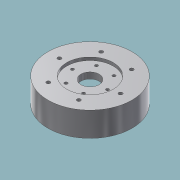
# Autodesk Inventor part: Spur Gear2
Saved by Autodesk Inventor 2017 SP1 (Build 210196100, 196)
## iProperties
Created: 2018-10-09
Part Number: Spur Gear2
Material: ABS Plastic
Document SubType Name: Modeling
Designer: Zach
Categories: <?xml version="1.0" encoding="UTF-16"?> <MemberInstance><Categories><FamilyTemplate><FamilyTemplateParameter ValueType="xs:double" Id="1" ObjectReferenceKey="da_z" ObjectType="kUserParameterObject"/><FamilyTemplateParameter ValueType="xs:double" Id="2" ObjectReferenceKey="da_b" ObjectType="kUserParameterObject"/><FamilyTemplateParameter ValueType="xs:double" Id="3" ObjectReferenceKey="da_beta" ObjectType="kUserParameterObject"/><FamilyTemplateParameter ValueType="xs:double" Id="4" ObjectReferenceKey="da_da" ObjectType="kUserParameterObject"/><FamilyTemplateParameter ValueType="xs:double" Id="5" ObjectReferenceKey="da_aw" ObjectType="kUserParameterObject"/><FamilyTemplateParameter ValueType="xs:string" Id="6" ObjectReferenceKey="EAIAABAAAACIAQAAAAAAAIAAAAAAAAAA" ObjectType="83910656" SubObjectId="SurfaceGeometry"/></FamilyTemplate><ParamToTemplateMap><ParamToTemplate CategoryParameter="//CategoryParameter[@InternalName='046C89C9-8512-4d59-83FE-43B91F4F132A']" TemplateParameter="1"/><ParamToTemplate CategoryParameter="//CategoryParameter[@InternalName='2552DF32-E462-4b46-AEBF-C6C7768E72AC']" TemplateParameter="2"/><ParamToTemplate CategoryParameter="//CategoryParameter[@InternalName='C9EE641D-15FC-4fae-A226-E94C4372FDD7']" TemplateParameter="3"/><ParamToTemplate><ParamToTemplate CategoryParameter="//CategoryParameter[@InternalName='00B6519A-459B-49c7-AD84-2E56D39A5744']" ConstantValue="0.000000"/></ParamToTemplate><ParamToTemplate><ParamToTemplate CategoryParameter="//CategoryParameter[@InternalName='04B31F0E-C7A6-4894-AA32-9629BEFACF47']" ConstantValue="1.000000"/></ParamToTemplate><ParamToTemplate><ParamToTemplate CategoryParameter="//CategoryParameter[@InternalName='43CBEC2E-7847-49e7-A936-2F7889FCB2D9']" ConstantValue="0.250000"/></ParamToTemplate><ParamToTemplate><ParamToTemplate CategoryParameter="//CategoryParameter[@InternalName='B1EFC894-105D-4ebd-86BF-FA20ED196853']" ConstantValue="0.350000"/></ParamToTemplate><ParamToTemplate><ParamToTemplate CategoryParameter="//CategoryParameter[@InternalName='51175063-3D10-4879-93E8-6246FE8B403D']" ConstantValue="2060000000.000000"/></ParamToTemplate><ParamToTemplate><ParamToTemplate CategoryParameter="//CategoryParameter[@InternalName='A3A52E27-4454-46a9-B0BD-C932399B70AF']" ConstantValue="0.300000"/></ParamToTemplate><ParamToTemplate><ParamToTemplate CategoryParameter="//CategoryParameter[@InternalName='91B76062-C214-41d9-B1B9-14D2AB99603D']" ConstantValue="0.200000"/></ParamToTemplate><ParamToTemplate><ParamToTemplate CategoryParameter="//CategoryParameter[@InternalName='374E806E-8B8A-4dda-A9AA-1039D6500AD2']" ConstantValue="5.000000"/></ParamToTemplate><ParamToTemplate><ParamToTemplate CategoryParameter="//CategoryParameter[@InternalName='2D373A89-B862-43d6-8D0B-0CBF12AB9F6C']" ConstantValue="0.392699"/></ParamToTemplate><ParamToTemplate CategoryParameter="//CategoryParameter[@InternalName='37777632-D6A2-4fac-9D53-DB8ACD95C989']" TemplateParameter="4"/><ParamToTemplate CategoryParameter="//CategoryParameter[@InternalName='FD1017F1-B727-4f7e-9707-0F86F1FF9423']" TemplateParameter="5"/><ParamToTemplate><ParamToTemplate CategoryParameter="//CategoryParameter[@InternalName='9E1B4470-B2D3-4ff1-B813-535BB4CDF51A']" ConstantValue="3520000.000000"/></ParamToTemplate><ParamToTemplate><ParamToTemplate CategoryParameter="//CategoryParameter[@InternalName='F8452263-BFF6-458c-9FB1-07C4B99E95CD']" ConstantValue="11400000.000000"/></ParamToTemplate><ParamToTemplate><ParamToTemplate CategoryParameter="//CategoryParameter[@InternalName='3E3BB259-FD49-497f-8171-6EBC954A3479']" ConstantValue="2.000000"/></ParamToTemplate><ParamToTemplate CategoryParameter="//CategoryParameter[@InternalName='27C3BAF2-7550-4e4b-AE2C-0DB134B7D9B7']" TemplateParameter="6"/></ParamToTemplateMap><Category DisplayName="Gear" InternalName="DC85795E-93AB-48d5-8EEE-5A27447B64BD" Mnemonic="Gear"><CategoryParameter DisplayName="z" InternalName="046C89C9-8512-4d59-83FE-43B91F4F132A" Mnemonic="z"/><CategoryParameter DisplayName="b" InternalName="2552DF32-E462-4b46-AEBF-C6C7768E72AC" Mnemonic="b"/><CategoryParameter DisplayName="||b|" InternalName="C9EE641D-15FC-4fae-A226-E94C4372FDD7" Mnemonic="beta"/><CategoryParameter DisplayName="x" InternalName="00B6519A-459B-49c7-AD84-2E56D39A5744" Mnemonic="x"/><CategoryParameter DisplayName="a*" InternalName="04B31F0E-C7A6-4894-AA32-9629BEFACF47" Mnemonic="a"/><CategoryParameter DisplayName="c*" InternalName="43CBEC2E-7847-49e7-A936-2F7889FCB2D9" Mnemonic="c"/><CategoryParameter DisplayName="r|.f|*" InternalName="B1EFC894-105D-4ebd-86BF-FA20ED196853" Mnemonic="rf"/><CategoryParameter DisplayName="E" InternalName="51175063-3D10-4879-93E8-6246FE8B403D" Mnemonic="E"/><CategoryParameter DisplayName="||m|" InternalName="A3A52E27-4454-46a9-B0BD-C932399B70AF" Mnemonic="mi"/><Category DisplayName="SpurGear" InternalName="26C5A22E-A91E-4dfd-A3B3-23CCAFAE1764" Mnemonic="SpurGear"><CategoryParameter DisplayName="m" InternalName="91B76062-C214-41d9-B1B9-14D2AB99603D" Mnemonic="m"/><CategoryParameter DisplayName="P" InternalName="374E806E-8B8A-4dda-A9AA-1039D6500AD2" Mnemonic="PP"/><CategoryParameter DisplayName="||a|" InternalName="2D373A89-B862-43d6-8D0B-0CBF12AB9F6C" Mnemonic="alpha"/><CategoryParameter DisplayName="d|.a|" InternalName="37777632-D6A2-4fac-9D53-DB8ACD95C989" Mnemonic="da"/><CategoryParameter DisplayName="a|.w|" InternalName="FD1017F1-B727-4f7e-9707-0F86F1FF9423" Mnemonic="aw"/><CategoryParameter DisplayName="||s||.Flim|" InternalName="9E1B4470-B2D3-4ff1-B813-535BB4CDF51A" Mnemonic="sFlim"/><CategoryParameter DisplayName="||s||.Hlim|" InternalName="F8452263-BFF6-458c-9FB1-07C4B99E95CD" Mnemonic="sHlim"/><CategoryParameter DisplayName="type" InternalName="3E3BB259-FD49-497f-8171-6EBC954A3479" Mnemonic="type"/><Category DisplayName="InternalSpurGear" InternalName="7CF704F6-14A9-42f8-93CE-E71DF57C2B55" Mnemonic="InternalSpurGear"><CategoryParameter DisplayName="PitchDiameter" InternalName="27C3BAF2-7550-4e4b-AE2C-0DB134B7D9B7" Mnemonic="IDS_PITCHDIAM"/></Category></Category></Category></Categories></MemberInstance>
Density: 1.06 g/cm^3
Appearance: Smooth - White
CustomPartVersion: 0
Author: Zach
Autodesk Inventor part; units mm, degrees
ref_plane "YZ Plane" through (0, 0, 0) normal (1, 0, 0) x (0, 1, 0)
ref_plane "XZ Plane" through (0, 0, 0) normal (0, 1, 0) x (-1, 0, 0)
ref_plane "XY Plane" through (0, 0, 0) normal (0, 0, 1) x (1, 0, 0)
sketch "Sketch1" plane through (0, 0, 0) normal (0, 0, 1) x (1, 0, 0)
  circle A0 centre (0, 0) radius 68.75
  dimension "d0" = 137.5
  constraints: 1 centre point
  measures "d0" diameter of A0
extrude "Extrusion1" add sketch "Sketch1" along normal blind 10
ref_plane "Work Plane2" through (0, 0, 5) normal (0, 0, 1) x (1, 0, 0)
sketch "Sketch2" plane through (0, 0, 0) normal (0, 0, -1) x (-1, 0, 0)
  circle A0 centre (0, 0) radius 68.75 projected
  circle A1 centre (0, 0) radius 60
  dimension "d3" = 120
  constraints: 1 centre point, 1 coincident
  measures "d3" diameter of A1
surface extrude "Pitch Diameter" sketch "Sketch2" against normal through all shown no curves A1
ref_plane "Work Plane8" through (0, 0, 0) normal (0.9986295, 0.052336, 0) x (0, 0, 1)
ref_plane "Work Plane9" through (0, 0, 0) normal (1, 0, 0) x (0, 1, 0)
spur gear teeth "Spur Gear" teeth 60 pitch diameter 120 tip diameter 116 root diameter 125 face width 10 start plane through (0, 0, 0) normal (0, 0, -1) x (-1, 0, 0)
sketch "Sketch3" plane through (0, 0, 10) normal (0, 0, 1) x (1, 0, 0)
  arc A0 (2.2771, -57.9553) -> (3.7934, -57.8758) centre (0, 0) ccw projected
  arc A1 (0.8181, -62.4946) -> (2.2771, -57.9553) centre (-22.2852, -52.565) ccw projected
  arc A2 (-0.8181, -62.4946) -> (0.8181, -62.4946) centre (0, 0) ccw projected
  arc A3 (-2.2771, -57.9553) -> (-0.8181, -62.4946) centre (22.2852, -52.565) ccw projected
  arc A4 (-3.7934, -57.8758) -> (-2.2771, -57.9553) centre (0, 0) ccw projected
  arc A5 (-5.7189, -62.2378) -> (-3.7934, -57.8758) centre (-27.6576, -49.9476) ccw projected
  arc A6 (-7.3461, -62.0668) -> (-5.7189, -62.2378) centre (0, 0) ccw projected
  arc A7 (-8.3226, -57.3998) -> (-7.3461, -62.0668) centre (16.6686, -54.6065) ccw projected
  arc A8 (-9.8223, -57.1623) -> (-8.3226, -57.3998) centre (0, 0) ccw projected
  arc A9 (-12.1931, -61.2991) -> (-9.8223, -57.1623) centre (-32.7271, -46.783) ccw projected
  arc A10 (-13.7936, -60.9589) -> (-12.1931, -61.2991) centre (0, 0) ccw projected
  arc A11 (-14.2769, -56.2154) -> (-13.7936, -60.9589) centre (10.8693, -56.0497) ccw projected
  arc A12 (-15.7435, -55.8224) -> (-14.2769, -56.2154) centre (0, 0) ccw projected
  arc A13 (-18.5338, -59.6887) -> (-15.7435, -55.8224) centre (-37.438, -43.1058) ccw projected
  arc A14 (-20.09, -59.1831) -> (-18.5338, -59.6887) centre (0, 0) ccw projected
  arc A15 (-20.0748, -54.4151) -> (-20.09, -59.1831) centre (4.951, -56.8788) ccw projected
  arc A16 (-21.4923, -53.871) -> (-20.0748, -54.4151) centre (0, 0) ccw projected
  arc A17 (-24.6715, -57.4245) -> (-21.4923, -53.871) centre (-41.7386, -38.9563) ccw projected
  arc A18 (-26.1662, -56.7589) -> (-24.6715, -57.4245) centre (0, 0) ccw projected
  arc A19 (-25.6527, -52.0186) -> (-26.1662, -56.7589) centre (-1.0216, -57.0847) ccw projected
  arc A20 (-27.0056, -51.3293) -> (-25.6527, -52.0186) centre (0, 0) ccw projected
  arc A21 (-30.5388, -54.531) -> (-27.0056, -51.3293) centre (-45.582, -34.38) ccw projected
  arc A22 (-31.9558, -53.7129) -> (-30.5388, -54.531) centre (0, 0) ccw projected
  arc A23 (-30.9496, -49.0522) -> (-31.9558, -53.7129) centre (-6.983, -56.6652) ccw projected
  arc A24 (-32.2231, -48.2252) -> (-30.9496, -49.0522) centre (0, 0) ccw projected
  arc A25 (-36.0716, -51.0401) -> (-32.2231, -48.2252) centre (-48.926, -29.4271) ccw projected
  arc A26 (-37.3953, -50.0784) -> (-36.0716, -51.0401) centre (0, 0) ccw projected
  arc A27 (-35.9074, -45.5484) -> (-37.3953, -50.0784) centre (-12.8678, -55.6249) ccw projected
  arc A28 (-37.0875, -44.5928) -> (-35.9074, -45.5484) centre (0, 0) ccw projected
  arc A29 (-41.2091, -46.99) -> (-37.0875, -44.5928) centre (-51.734, -24.1517) ccw projected
  arc A30 (-42.425, -45.8952) -> (-41.2091, -46.99) centre (0, 0) ccw projected
  arc A31 (-40.4718, -41.5455) -> (-42.425, -45.8952) centre (-18.6117, -53.9751) ccw projected
  arc A32 (-41.5455, -40.4718) -> (-40.4718, -41.5455) centre (0, 0) ccw projected
  arc A33 (-45.8952, -42.425) -> (-41.5455, -40.4718) centre (-53.9751, -18.6117) ccw projected
  arc A34 (-46.99, -41.2091) -> (-45.8952, -42.425) centre (0, 0) ccw projected
  arc A35 (-44.5928, -37.0875) -> (-46.99, -41.2091) centre (-24.1517, -51.734) ccw projected
  arc A36 (-45.5484, -35.9074) -> (-44.5928, -37.0875) centre (0, 0) ccw projected
  arc A37 (-50.0784, -37.3953) -> (-45.5484, -35.9074) centre (-55.6249, -12.8678) ccw projected
  arc A38 (-51.0401, -36.0716) -> (-50.0784, -37.3953) centre (0, 0) ccw projected
  arc A39 (-48.2252, -32.2231) -> (-51.0401, -36.0716) centre (-29.4271, -48.926) ccw projected
  arc A40 (-49.0522, -30.9496) -> (-48.2252, -32.2231) centre (0, 0) ccw projected
  arc A41 (-53.7129, -31.9558) -> (-49.0522, -30.9496) centre (-56.6652, -6.983) ccw projected
  arc A42 (-54.531, -30.5388) -> (-53.7129, -31.9558) centre (0, 0) ccw projected
  arc A43 (-51.3293, -27.0056) -> (-54.531, -30.5388) centre (-34.38, -45.582) ccw projected
  arc A44 (-52.0186, -25.6527) -> (-51.3293, -27.0056) centre (0, 0) ccw projected
  arc A45 (-56.7589, -26.1662) -> (-52.0186, -25.6527) centre (-57.0847, -1.0216) ccw projected
  arc A46 (-57.4245, -24.6715) -> (-56.7589, -26.1662) centre (0, 0) ccw projected
  arc A47 (-53.871, -21.4923) -> (-57.4245, -24.6715) centre (-38.9563, -41.7386) ccw projected
  arc A48 (-54.4151, -20.0748) -> (-53.871, -21.4923) centre (0, 0) ccw projected
  arc A49 (-59.1831, -20.09) -> (-54.4151, -20.0748) centre (-56.8788, 4.951) ccw projected
  arc A50 (-59.6887, -18.5338) -> (-59.1831, -20.09) centre (0, 0) ccw projected
  arc A51 (-55.8224, -15.7435) -> (-59.6887, -18.5338) centre (-43.1058, -37.438) ccw projected
  arc A52 (-56.2154, -14.2769) -> (-55.8224, -15.7435) centre (0, 0) ccw projected
  arc A53 (-60.9589, -13.7936) -> (-56.2154, -14.2769) centre (-56.0497, 10.8693) ccw projected
  arc A54 (-61.2991, -12.1931) -> (-60.9589, -13.7936) centre (0, 0) ccw projected
  arc A55 (-57.1623, -9.8223) -> (-61.2991, -12.1931) centre (-46.783, -32.7271) ccw projected
  arc A56 (-57.3998, -8.3226) -> (-57.1623, -9.8223) centre (0, 0) ccw projected
  arc A57 (-62.0668, -7.3461) -> (-57.3998, -8.3226) centre (-54.6065, 16.6686) ccw projected
  arc A58 (-62.2378, -5.7189) -> (-62.0668, -7.3461) centre (0, 0) ccw projected
  arc A59 (-57.8758, -3.7934) -> (-62.2378, -5.7189) centre (-49.9476, -27.6576) ccw projected
  arc A60 (-57.9553, -2.2771) -> (-57.8758, -3.7934) centre (0, 0) ccw projected
  arc A61 (-62.4946, -0.8181) -> (-57.9553, -2.2771) centre (-52.565, 22.2852) ccw projected
  arc A62 (-62.4946, 0.8181) -> (-62.4946, -0.8181) centre (0, 0) ccw projected
  arc A63 (-57.9553, 2.2771) -> (-62.4946, 0.8181) centre (-52.565, -22.2852) ccw projected
  arc A64 (-57.8758, 3.7934) -> (-57.9553, 2.2771) centre (0, 0) ccw projected
  arc A65 (-62.2378, 5.7189) -> (-57.8758, 3.7934) centre (-49.9476, 27.6576) ccw projected
  arc A66 (-62.0668, 7.3461) -> (-62.2378, 5.7189) centre (0, 0) ccw projected
  arc A67 (-57.3998, 8.3226) -> (-62.0668, 7.3461) centre (-54.6065, -16.6686) ccw projected
  arc A68 (-57.1623, 9.8223) -> (-57.3998, 8.3226) centre (0, 0) ccw projected
  arc A69 (-61.2991, 12.1931) -> (-57.1623, 9.8223) centre (-46.783, 32.7271) ccw projected
  arc A70 (-60.9589, 13.7936) -> (-61.2991, 12.1931) centre (0, 0) ccw projected
  arc A71 (-56.2154, 14.2769) -> (-60.9589, 13.7936) centre (-56.0497, -10.8693) ccw projected
  arc A72 (-55.8224, 15.7435) -> (-56.2154, 14.2769) centre (0, 0) ccw projected
  arc A73 (-59.6887, 18.5338) -> (-55.8224, 15.7435) centre (-43.1058, 37.438) ccw projected
  arc A74 (-59.1831, 20.09) -> (-59.6887, 18.5338) centre (0, 0) ccw projected
  arc A75 (-54.4151, 20.0748) -> (-59.1831, 20.09) centre (-56.8788, -4.951) ccw projected
  arc A76 (-53.871, 21.4923) -> (-54.4151, 20.0748) centre (0, 0) ccw projected
  arc A77 (-57.4245, 24.6715) -> (-53.871, 21.4923) centre (-38.9563, 41.7386) ccw projected
  arc A78 (-56.7589, 26.1662) -> (-57.4245, 24.6715) centre (0, 0) ccw projected
  arc A79 (-52.0186, 25.6527) -> (-56.7589, 26.1662) centre (-57.0847, 1.0216) ccw projected
  arc A80 (-51.3293, 27.0056) -> (-52.0186, 25.6527) centre (0, 0) ccw projected
  arc A81 (-54.531, 30.5388) -> (-51.3293, 27.0056) centre (-34.38, 45.582) ccw projected
  arc A82 (-53.7129, 31.9558) -> (-54.531, 30.5388) centre (0, 0) ccw projected
  arc A83 (-49.0522, 30.9496) -> (-53.7129, 31.9558) centre (-56.6652, 6.983) ccw projected
  arc A84 (-48.2252, 32.2231) -> (-49.0522, 30.9496) centre (0, 0) ccw projected
  arc A85 (-51.0401, 36.0716) -> (-48.2252, 32.2231) centre (-29.4271, 48.926) ccw projected
  arc A86 (-50.0784, 37.3953) -> (-51.0401, 36.0716) centre (0, 0) ccw projected
  arc A87 (-45.5484, 35.9074) -> (-50.0784, 37.3953) centre (-55.6249, 12.8678) ccw projected
  arc A88 (-44.5928, 37.0875) -> (-45.5484, 35.9074) centre (0, 0) ccw projected
  arc A89 (-46.99, 41.2091) -> (-44.5928, 37.0875) centre (-24.1517, 51.734) ccw projected
  arc A90 (-45.8952, 42.425) -> (-46.99, 41.2091) centre (0, 0) ccw projected
  arc A91 (-41.5455, 40.4718) -> (-45.8952, 42.425) centre (-53.9751, 18.6117) ccw projected
  arc A92 (-40.4718, 41.5455) -> (-41.5455, 40.4718) centre (0, 0) ccw projected
  arc A93 (-42.425, 45.8952) -> (-40.4718, 41.5455) centre (-18.6117, 53.9751) ccw projected
  arc A94 (-41.2091, 46.99) -> (-42.425, 45.8952) centre (0, 0) ccw projected
  arc A95 (-37.0875, 44.5928) -> (-41.2091, 46.99) centre (-51.734, 24.1517) ccw projected
  arc A96 (-35.9074, 45.5484) -> (-37.0875, 44.5928) centre (0, 0) ccw projected
  arc A97 (-37.3953, 50.0784) -> (-35.9074, 45.5484) centre (-12.8678, 55.6249) ccw projected
  arc A98 (-36.0716, 51.0401) -> (-37.3953, 50.0784) centre (0, 0) ccw projected
  arc A99 (-32.2231, 48.2252) -> (-36.0716, 51.0401) centre (-48.926, 29.4271) ccw projected
  arc A100 (-30.9496, 49.0522) -> (-32.2231, 48.2252) centre (0, 0) ccw projected
  arc A101 (-31.9558, 53.7129) -> (-30.9496, 49.0522) centre (-6.983, 56.6652) ccw projected
  arc A102 (-30.5388, 54.531) -> (-31.9558, 53.7129) centre (0, 0) ccw projected
  arc A103 (-27.0056, 51.3293) -> (-30.5388, 54.531) centre (-45.582, 34.38) ccw projected
  arc A104 (-25.6527, 52.0186) -> (-27.0056, 51.3293) centre (0, 0) ccw projected
  arc A105 (-26.1662, 56.7589) -> (-25.6527, 52.0186) centre (-1.0216, 57.0847) ccw projected
  arc A106 (-24.6715, 57.4245) -> (-26.1662, 56.7589) centre (0, 0) ccw projected
  arc A107 (-21.4923, 53.871) -> (-24.6715, 57.4245) centre (-41.7386, 38.9563) ccw projected
  arc A108 (-20.0748, 54.4151) -> (-21.4923, 53.871) centre (0, 0) ccw projected
  arc A109 (-20.09, 59.1831) -> (-20.0748, 54.4151) centre (4.951, 56.8788) ccw projected
  arc A110 (-18.5338, 59.6887) -> (-20.09, 59.1831) centre (0, 0) ccw projected
  arc A111 (-15.7435, 55.8224) -> (-18.5338, 59.6887) centre (-37.438, 43.1058) ccw projected
  arc A112 (-14.2769, 56.2154) -> (-15.7435, 55.8224) centre (0, 0) ccw projected
  arc A113 (-13.7936, 60.9589) -> (-14.2769, 56.2154) centre (10.8693, 56.0497) ccw projected
  arc A114 (-12.1931, 61.2991) -> (-13.7936, 60.9589) centre (0, 0) ccw projected
  arc A115 (-9.8223, 57.1623) -> (-12.1931, 61.2991) centre (-32.7271, 46.783) ccw projected
  arc A116 (-8.3226, 57.3998) -> (-9.8223, 57.1623) centre (0, 0) ccw projected
  arc A117 (-7.3461, 62.0668) -> (-8.3226, 57.3998) centre (16.6686, 54.6065) ccw projected
  arc A118 (-5.7189, 62.2378) -> (-7.3461, 62.0668) centre (0, 0) ccw projected
  arc A119 (-3.7934, 57.8758) -> (-5.7189, 62.2378) centre (-27.6576, 49.9476) ccw projected
  arc A120 (-2.2771, 57.9553) -> (-3.7934, 57.8758) centre (0, 0) ccw projected
  arc A121 (-0.8181, 62.4946) -> (-2.2771, 57.9553) centre (22.2852, 52.565) ccw projected
  arc A122 (0.8181, 62.4946) -> (-0.8181, 62.4946) centre (0, 0) ccw projected
  arc A123 (2.2771, 57.9553) -> (0.8181, 62.4946) centre (-22.2852, 52.565) ccw projected
  arc A124 (3.7934, 57.8758) -> (2.2771, 57.9553) centre (0, 0) ccw projected
  arc A125 (5.7189, 62.2378) -> (3.7934, 57.8758) centre (27.6576, 49.9476) ccw projected
  arc A126 (7.3461, 62.0668) -> (5.7189, 62.2378) centre (0, 0) ccw projected
  arc A127 (8.3226, 57.3998) -> (7.3461, 62.0668) centre (-16.6686, 54.6065) ccw projected
  arc A128 (9.8223, 57.1623) -> (8.3226, 57.3998) centre (0, 0) ccw projected
  arc A129 (12.1931, 61.2991) -> (9.8223, 57.1623) centre (32.7271, 46.783) ccw projected
  arc A130 (13.7936, 60.9589) -> (12.1931, 61.2991) centre (0, 0) ccw projected
  arc A131 (14.2769, 56.2154) -> (13.7936, 60.9589) centre (-10.8693, 56.0497) ccw projected
  arc A132 (15.7435, 55.8224) -> (14.2769, 56.2154) centre (0, 0) ccw projected
  arc A133 (18.5338, 59.6887) -> (15.7435, 55.8224) centre (37.438, 43.1058) ccw projected
  arc A134 (20.09, 59.1831) -> (18.5338, 59.6887) centre (0, 0) ccw projected
  arc A135 (20.0748, 54.4151) -> (20.09, 59.1831) centre (-4.951, 56.8788) ccw projected
  arc A136 (21.4923, 53.871) -> (20.0748, 54.4151) centre (0, 0) ccw projected
  arc A137 (24.6715, 57.4245) -> (21.4923, 53.871) centre (41.7386, 38.9563) ccw projected
  arc A138 (26.1662, 56.7589) -> (24.6715, 57.4245) centre (0, 0) ccw projected
  arc A139 (25.6527, 52.0186) -> (26.1662, 56.7589) centre (1.0216, 57.0847) ccw projected
  arc A140 (27.0056, 51.3293) -> (25.6527, 52.0186) centre (0, 0) ccw projected
  arc A141 (30.5388, 54.531) -> (27.0056, 51.3293) centre (45.582, 34.38) ccw projected
  arc A142 (31.9558, 53.7129) -> (30.5388, 54.531) centre (0, 0) ccw projected
  arc A143 (30.9496, 49.0522) -> (31.9558, 53.7129) centre (6.983, 56.6652) ccw projected
  arc A144 (32.2231, 48.2252) -> (30.9496, 49.0522) centre (0, 0) ccw projected
  arc A145 (36.0716, 51.0401) -> (32.2231, 48.2252) centre (48.926, 29.4271) ccw projected
  arc A146 (37.3953, 50.0784) -> (36.0716, 51.0401) centre (0, 0) ccw projected
  arc A147 (35.9074, 45.5484) -> (37.3953, 50.0784) centre (12.8678, 55.6249) ccw projected
  arc A148 (37.0875, 44.5928) -> (35.9074, 45.5484) centre (0, 0) ccw projected
  arc A149 (41.2091, 46.99) -> (37.0875, 44.5928) centre (51.734, 24.1517) ccw projected
  arc A150 (42.425, 45.8952) -> (41.2091, 46.99) centre (0, 0) ccw projected
  arc A151 (40.4718, 41.5455) -> (42.425, 45.8952) centre (18.6117, 53.9751) ccw projected
  arc A152 (41.5455, 40.4718) -> (40.4718, 41.5455) centre (0, 0) ccw projected
  arc A153 (45.8952, 42.425) -> (41.5455, 40.4718) centre (53.9751, 18.6117) ccw projected
  arc A154 (46.99, 41.2091) -> (45.8952, 42.425) centre (0, 0) ccw projected
  arc A155 (44.5928, 37.0875) -> (46.99, 41.2091) centre (24.1517, 51.734) ccw projected
  arc A156 (45.5484, 35.9074) -> (44.5928, 37.0875) centre (0, 0) ccw projected
  arc A157 (50.0784, 37.3953) -> (45.5484, 35.9074) centre (55.6249, 12.8678) ccw projected
  arc A158 (51.0401, 36.0716) -> (50.0784, 37.3953) centre (0, 0) ccw projected
  arc A159 (48.2252, 32.2231) -> (51.0401, 36.0716) centre (29.4271, 48.926) ccw projected
  arc A160 (49.0522, 30.9496) -> (48.2252, 32.2231) centre (0, 0) ccw projected
  arc A161 (53.7129, 31.9558) -> (49.0522, 30.9496) centre (56.6652, 6.983) ccw projected
  arc A162 (54.531, 30.5388) -> (53.7129, 31.9558) centre (0, 0) ccw projected
  arc A163 (51.3293, 27.0056) -> (54.531, 30.5388) centre (34.38, 45.582) ccw projected
  arc A164 (52.0186, 25.6527) -> (51.3293, 27.0056) centre (0, 0) ccw projected
  arc A165 (56.7589, 26.1662) -> (52.0186, 25.6527) centre (57.0847, 1.0216) ccw projected
  arc A166 (57.4245, 24.6715) -> (56.7589, 26.1662) centre (0, 0) ccw projected
  arc A167 (53.871, 21.4923) -> (57.4245, 24.6715) centre (38.9563, 41.7386) ccw projected
  arc A168 (54.4151, 20.0748) -> (53.871, 21.4923) centre (0, 0) ccw projected
  arc A169 (59.1831, 20.09) -> (54.4151, 20.0748) centre (56.8788, -4.951) ccw projected
  arc A170 (59.6887, 18.5338) -> (59.1831, 20.09) centre (0, 0) ccw projected
  arc A171 (55.8224, 15.7435) -> (59.6887, 18.5338) centre (43.1058, 37.438) ccw projected
  arc A172 (56.2154, 14.2769) -> (55.8224, 15.7435) centre (0, 0) ccw projected
  arc A173 (60.9589, 13.7936) -> (56.2154, 14.2769) centre (56.0497, -10.8693) ccw projected
  arc A174 (61.2991, 12.1931) -> (60.9589, 13.7936) centre (0, 0) ccw projected
  arc A175 (57.1623, 9.8223) -> (61.2991, 12.1931) centre (46.783, 32.7271) ccw projected
  arc A176 (57.3998, 8.3226) -> (57.1623, 9.8223) centre (0, 0) ccw projected
  arc A177 (62.0668, 7.3461) -> (57.3998, 8.3226) centre (54.6065, -16.6686) ccw projected
  arc A178 (62.2378, 5.7189) -> (62.0668, 7.3461) centre (0, 0) ccw projected
  arc A179 (57.8758, 3.7934) -> (62.2378, 5.7189) centre (49.9476, 27.6576) ccw projected
  arc A180 (57.9553, 2.2771) -> (57.8758, 3.7934) centre (0, 0) ccw projected
  arc A181 (62.4946, 0.8181) -> (57.9553, 2.2771) centre (52.565, -22.2852) ccw projected
  arc A182 (62.4946, -0.8181) -> (62.4946, 0.8181) centre (0, 0) ccw projected
  arc A183 (57.9553, -2.2771) -> (62.4946, -0.8181) centre (52.565, 22.2852) ccw projected
  arc A184 (57.8758, -3.7934) -> (57.9553, -2.2771) centre (0, 0) ccw projected
  arc A185 (62.2378, -5.7189) -> (57.8758, -3.7934) centre (49.9476, -27.6576) ccw projected
  arc A186 (62.0668, -7.3461) -> (62.2378, -5.7189) centre (0, 0) ccw projected
  arc A187 (57.3998, -8.3226) -> (62.0668, -7.3461) centre (54.6065, 16.6686) ccw projected
  arc A188 (57.1623, -9.8223) -> (57.3998, -8.3226) centre (0, 0) ccw projected
  arc A189 (61.2991, -12.1931) -> (57.1623, -9.8223) centre (46.783, -32.7271) ccw projected
  arc A190 (60.9589, -13.7936) -> (61.2991, -12.1931) centre (0, 0) ccw projected
  arc A191 (56.2154, -14.2769) -> (60.9589, -13.7936) centre (56.0497, 10.8693) ccw projected
  arc A192 (55.8224, -15.7435) -> (56.2154, -14.2769) centre (0, 0) ccw projected
  arc A193 (59.6887, -18.5338) -> (55.8224, -15.7435) centre (43.1058, -37.438) ccw projected
  arc A194 (59.1831, -20.09) -> (59.6887, -18.5338) centre (0, 0) ccw projected
  arc A195 (54.4151, -20.0748) -> (59.1831, -20.09) centre (56.8788, 4.951) ccw projected
  arc A196 (53.871, -21.4923) -> (54.4151, -20.0748) centre (0, 0) ccw projected
  arc A197 (57.4245, -24.6715) -> (53.871, -21.4923) centre (38.9563, -41.7386) ccw projected
  arc A198 (56.7589, -26.1662) -> (57.4245, -24.6715) centre (0, 0) ccw projected
  arc A199 (52.0186, -25.6527) -> (56.7589, -26.1662) centre (57.0847, -1.0216) ccw projected
  arc A200 (51.3293, -27.0056) -> (52.0186, -25.6527) centre (0, 0) ccw projected
  arc A201 (54.531, -30.5388) -> (51.3293, -27.0056) centre (34.38, -45.582) ccw projected
  arc A202 (53.7129, -31.9558) -> (54.531, -30.5388) centre (0, 0) ccw projected
  arc A203 (49.0522, -30.9496) -> (53.7129, -31.9558) centre (56.6652, -6.983) ccw projected
  arc A204 (48.2252, -32.2231) -> (49.0522, -30.9496) centre (0, 0) ccw projected
  arc A205 (51.0401, -36.0716) -> (48.2252, -32.2231) centre (29.4271, -48.926) ccw projected
  arc A206 (50.0784, -37.3953) -> (51.0401, -36.0716) centre (0, 0) ccw projected
  arc A207 (45.5484, -35.9074) -> (50.0784, -37.3953) centre (55.6249, -12.8678) ccw projected
  arc A208 (44.5928, -37.0875) -> (45.5484, -35.9074) centre (0, 0) ccw projected
  arc A209 (46.99, -41.2091) -> (44.5928, -37.0875) centre (24.1517, -51.734) ccw projected
  arc A210 (45.8952, -42.425) -> (46.99, -41.2091) centre (0, 0) ccw projected
  arc A211 (41.5455, -40.4718) -> (45.8952, -42.425) centre (53.9751, -18.6117) ccw projected
  arc A212 (40.4718, -41.5455) -> (41.5455, -40.4718) centre (0, 0) ccw projected
  arc A213 (42.425, -45.8952) -> (40.4718, -41.5455) centre (18.6117, -53.9751) ccw projected
  arc A214 (41.2091, -46.99) -> (42.425, -45.8952) centre (0, 0) ccw projected
  arc A215 (37.0875, -44.5928) -> (41.2091, -46.99) centre (51.734, -24.1517) ccw projected
  arc A216 (35.9074, -45.5484) -> (37.0875, -44.5928) centre (0, 0) ccw projected
  arc A217 (37.3953, -50.0784) -> (35.9074, -45.5484) centre (12.8678, -55.6249) ccw projected
  arc A218 (36.0716, -51.0401) -> (37.3953, -50.0784) centre (0, 0) ccw projected
  arc A219 (32.2231, -48.2252) -> (36.0716, -51.0401) centre (48.926, -29.4271) ccw projected
  arc A220 (30.9496, -49.0522) -> (32.2231, -48.2252) centre (0, 0) ccw projected
  arc A221 (31.9558, -53.7129) -> (30.9496, -49.0522) centre (6.983, -56.6652) ccw projected
  arc A222 (30.5388, -54.531) -> (31.9558, -53.7129) centre (0, 0) ccw projected
  arc A223 (27.0056, -51.3293) -> (30.5388, -54.531) centre (45.582, -34.38) ccw projected
  arc A224 (25.6527, -52.0186) -> (27.0056, -51.3293) centre (0, 0) ccw projected
  arc A225 (26.1662, -56.7589) -> (25.6527, -52.0186) centre (1.0216, -57.0847) ccw projected
  arc A226 (24.6715, -57.4245) -> (26.1662, -56.7589) centre (0, 0) ccw projected
  arc A227 (21.4923, -53.871) -> (24.6715, -57.4245) centre (41.7386, -38.9563) ccw projected
  arc A228 (20.0748, -54.4151) -> (21.4923, -53.871) centre (0, 0) ccw projected
  arc A229 (20.09, -59.1831) -> (20.0748, -54.4151) centre (-4.951, -56.8788) ccw projected
  arc A230 (18.5338, -59.6887) -> (20.09, -59.1831) centre (0, 0) ccw projected
  arc A231 (15.7435, -55.8224) -> (18.5338, -59.6887) centre (37.438, -43.1058) ccw projected
  arc A232 (14.2769, -56.2154) -> (15.7435, -55.8224) centre (0, 0) ccw projected
  arc A233 (13.7936, -60.9589) -> (14.2769, -56.2154) centre (-10.8693, -56.0497) ccw projected
  arc A234 (12.1931, -61.2991) -> (13.7936, -60.9589) centre (0, 0) ccw projected
  arc A235 (9.8223, -57.1623) -> (12.1931, -61.2991) centre (32.7271, -46.783) ccw projected
  arc A236 (8.3226, -57.3998) -> (9.8223, -57.1623) centre (0, 0) ccw projected
  arc A237 (7.3461, -62.0668) -> (8.3226, -57.3998) centre (-16.6686, -54.6065) ccw projected
  arc A238 (5.7189, -62.2378) -> (7.3461, -62.0668) centre (0, 0) ccw projected
  arc A239 (3.7934, -57.8758) -> (5.7189, -62.2378) centre (27.6576, -49.9476) ccw projected
  circle A240 centre (0, 0) radius 68.75 projected
extrude "Extrusion2" add sketch "Sketch3" along normal blind 15
sketch "Sketch4" plane through (0, 0, 25) normal (0, 0, 1) x (1, 0, 0)
  circle A0 centre (0, 0) radius 68.75 projected
  circle A1 centre (0, 0) radius 15
  circle A2 centre (50, 0) radius 3
  circle A3 centre (25, 43.3013) radius 3
  circle A4 centre (-25, 43.3013) radius 3
  circle A5 centre (-50, 0) radius 3
  circle A6 centre (-25, -43.3013) radius 3
  circle A7 centre (25, -43.3013) radius 3
  dimension "d55" = 30
  dimension "d56" = 6
  dimension "d57" = 50
  dimension "d60" = 360
  constraints: 7 centre point, 1 coincident, 1 horizontal alignment, 13 other
  measures "d55" diameter of A1
  measures "d56" diameter of A2
  measures "d57" distance of A2.centre point (0, 0)
extrude "Extrusion3" add sketch "Sketch4" along normal blind 10
sketch "Sketch8" plane through (0, 0, 35) normal (0, 0, 1) x (1, 0, 0)
  circle A0 centre (-28.75, 0) radius 2.5
  circle A1 centre (0, 0) radius 20
  line L0 (-20, 0) -> (-37.5, 0) construction
  circle A2 centre (0, 0) radius 37.5
  circle A3 centre (-14.375, -24.8982) radius 2.5
  circle A4 centre (14.375, -24.8982) radius 2.5
  circle A5 centre (28.75, 0) radius 2.5
  circle A6 centre (14.375, 24.8982) radius 2.5
  circle A7 centre (-14.375, 24.8982) radius 2.5
  dimension "d70" = 5
  dimension "d73" = 360
  constraints: 6 centre point, 4 horizontal alignment, 2 end point, 1 coincident, 1 horizontal, 1 midpoint, 17 other
  measures "d70" diameter of A0
extrude "Extrusion6" cut sketch "Sketch8" against normal blind 10 contours A0 | A3 | A4 | A5 | A6 | A7
sketch "Sketch9" plane through (0, 0, 35) normal (0, 0, 1) x (1, 0, 0)
  circle A0 centre (0, 0) radius 38
  circle A1 centre (0, 0) radius 68.75 projected
  circle A2 centre (25, -43.3013) radius 3 projected
  circle A3 centre (50, 0) radius 3 projected
  circle A4 centre (25, 43.3013) radius 3 projected
  circle A5 centre (-25, 43.3013) radius 3 projected
  circle A6 centre (-50, 0) radius 3 projected
  circle A7 centre (-25, -43.3013) radius 3 projected
  dimension "d77" = 76
  constraints: 1 centre point, 1 coincident
  measures "d77" diameter of A0
extrude "Extrusion7" add sketch "Sketch9" along normal blind 5
equation "\"d0\" = 1.1 * da_df"
equation "\"d1\" = da_b"
equation "\"d3\" = da_dw"
equation "\"d16\" = da_aw"
equation "\"da_df\" = 125"
equation "\"da_b\" = 10"
equation "\"da_dw\" = 120"
equation "\"da_aw\" = 40"
body "Solid1"
body "Srf1"
